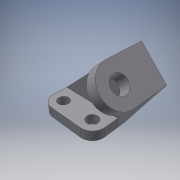
# Autodesk Inventor part: 스터디캐드캠 - 3D 모델링 연습도면 540
Saved by Autodesk Inventor 2017 (Build 210142000, 142)
## iProperties
Created: 2016-06-13
Part Number: 스터디캐드캠 - 3D 모델링 연습도면 540
Material: Generic
Document SubType Name: Modeling
Designer: Dibujo
Density: 1 g/cm^3
Appearance: Default
Mass: 60.4335 g
Surface Area: 174.131 cm^2
Volume: 60.4335 cm^3
Author: Dibujo
Autodesk Inventor part; units mm, degrees
note: some values were not read from the file. Chosen so that the rebuilt part matches the saved one: direction of "구멍1".
ref_plane "YZ Plane" through (0, 0, 0) normal (1, 0, 0) x (0, 1, 0)
ref_plane "XZ Plane" through (0, 0, 0) normal (0, 1, 0) x (-1, 0, 0)
ref_plane "XY Plane" through (0, 0, 0) normal (0, 0, 1) x (1, 0, 0)
sketch "Sketch1" plane through (0, 0, 0) normal (0, 1, 0) x (-1, 0, 0)
  arc A0 (-34, 13) -> (-47, 0) centre (-34, 0) ccw
  arc A1 (13, 0) -> (0, 13) centre (0, 0) ccw
  line L0 (0, 13) -> (-34, 13)
  line L1 (13, 0) -> (13, -25)
  line L2 (13, -25) -> (-47, -25)
  line L3 (-47, -25) -> (-47, 0)
  dimension "d25" = 60
  dimension "d26" = 13
  dimension "d27" = 13
  dimension "d28" = 25
  constraints: 8 end point, 4 point on circle, 4 tangent, 2 centre point, 2 perpendicular, 2 vertical, 1 coincident
  measures "d25" distance of L1.end L2.end
  measures "d26" radius of A0
  measures "d27" radius of A1
  measures "d28" distance from line of L2 A1.centre
extrude "Extrusion1" add sketch "Sketch1" along normal blind 10
sketch "Sketch2" plane through (0, 10, 0) normal (0, 1, 0) x (1, 0, 0)
  arc A0 (-13, 0) -> (0, -13) centre (0, 0) ccw projected
  arc A1 (34, -13) -> (47, 0) centre (34, 0) ccw projected
  circle A2 centre (0, 0) radius 6
  circle A3 centre (34, 0) radius 6
  dimension "d29" = 12
  constraints: 2 centre point, 2 coincident, 1 equal radius
  measures "d29" diameter of A3
extrude "Extrusion2" cut sketch "Sketch2" against normal blind 9.525
sketch "Sketch3" plane through (47, 0, -25) normal (0, 0, -1) x (-1, 0, 0)
  line L0 (0, 10) -> (60, 10) projected
  line L1 (0, 0) -> (0, 10) projected
  line L2 (-19.6162, 62.4195) -> (-7.3912, 75.0789)
  line L3 (-19.6162, 62.4195) -> (-30.6439, 51)
  line L4 (-30.6439, 51) -> (0, 0)
  line L5 (-7.3912, 75.0789) -> (60, 10)
  line L6 (0, 0) -> (0, 10)
  line L7 (60, 10) -> (0, 10)
  point P0 (47, 0)
  dimension "d30" = 44
  dimension "d31" = 90
  dimension "d32" = 51
  dimension "d33" = 105
  constraints: 12 end point, 3 collinear
  measures "d30" angle of L5 L0
  measures "d31" angle of L2 L5
  measures "d32" vertical distance of L3.end L1.start
  measures "d33" angle of L4 L3
extrude "Extrusion3" add sketch "Sketch3" against normal blind 10
sketch "Sketch4" plane through (54.3912, 75.0789, -25) normal (0.7193398, 0.6946584, 0) x (-0.6946584, 0.7193398, 0)
  line L0 (0, 0) -> (-33.4736, 0) projected
  line L1 (0, 0) -> (0, 10) projected
  line L2 (-33.4736, 10) -> (0, 10) projected
  line L3 (-33.4736, 0) -> (-33.4736, 10) projected
  arc A0 (0, 35) -> (-33.4736, 35) centre (-16.7368, 35) ccw
  line L4 (-33.4736, 35) -> (-33.4736, 0)
  line L5 (-33.4736, 0) -> (0, 0)
  line L6 (0, 0) -> (0, 35)
  point P0 (-16.224, 25)
  dimension "d34" = 35
  constraints: 6 end point, 2 collinear, 2 point on circle, 2 tangent, 1 centre point, 1 perpendicular
  measures "d34" distance from line of A0.centre L0
extrude "Extrusion4" add sketch "Sketch4" against normal blind 10 contours L2 L4 A0 L6
hole "구멍1" at (66.0175, 63.0394, 10) direction (-0.7193398, -0.6946584, 0) diameter 15 end up to surface
body "Solid1"
